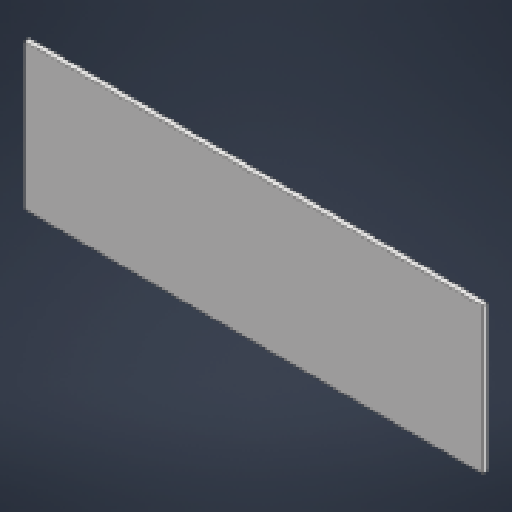
# Autodesk Inventor part: 挡板
Saved by Autodesk Inventor 2025 (Build 290162000, 162)
## iProperties
Created: 2024-12-26
Part Number: 挡板
Material: 常规
Document SubType Name: Modeling
Designer: HZD
Density: 1 g/cm^3
Appearance: 默认
Author: HZD
Autodesk Inventor part; units mm, degrees
ref_plane "YZ Plane" through (0, 0, 0) normal (1, 0, 0) x (0, 1, 0)
ref_plane "XZ Plane" through (0, 0, 0) normal (0, 1, 0) x (-1, 0, 0)
ref_plane "XY Plane" through (0, 0, 0) normal (0, 0, 1) x (1, 0, 0)
sketch "草图1" plane through (0, 0, 0) normal (0, 0, 1) x (1, 0, 0)
  line L0 (132.5, -42.1193) -> (-132.5, -42.1193)
  line L1 (-132.5, -42.1193) -> (-132.5, 42.1193)
  line L2 (-132.5, 42.1193) -> (132.5, 42.1193)
  line L3 (132.5, 42.1193) -> (132.5, -42.1193)
  line L4 (132.5, -42.1193) -> (-132.5, 42.1193) construction
  line L5 (-132.5, -42.1193) -> (132.5, 42.1193) construction
  point P0 (0, 0)
  dimension "d5" = 265
  constraints: 12 end point, 2 midpoint, 2 parallel, 1 horizontal, 1 perpendicular
  measures "d5" distance of L1.end L2.end
extrude "拉伸1" add sketch "草图1" along normal blind 3
